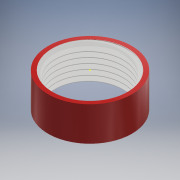
# Autodesk Inventor part: Rosca22
Saved by Autodesk Inventor 2018 (Build 220112000, 112)
## iProperties
Created: 2020-01-17
Part Number: Rosca22
Material: Generic
Document SubType Name: Modeling
Designer: Ivan
Density: 1 g/cm^3
Appearance: Default
Author: Ivan
Autodesk Inventor part; units mm, degrees
ref_plane "YZ Plane" through (0, 0, 0) normal (1, 0, 0) x (0, 1, 0)
ref_plane "XZ Plane" through (0, 0, 0) normal (0, 1, 0) x (-1, 0, 0)
ref_plane "XY Plane" through (0, 0, 0) normal (0, 0, 1) x (1, 0, 0)
sketch "Sketch1" plane through (0, 0, 0) normal (0, 0, 1) x (1, 0, 0)
  circle A0 centre (0, 0) radius 12.25
  dimension "d0" = 24.5
  constraints: 1 centre point, 1 coincident
  measures "d0" diameter of A0
extrude "Extrusion1" add sketch "Sketch1" along normal blind 10
sketch "Sketch2" plane through (0, 0, 10) normal (0, 0, 1) x (1, 0, 0)
  point P0 (0, 0)
sketch "Sketch3" plane through (0, 0, 10) normal (0, 0, 1) x (1, 0, 0)
  circle A0 centre (0, 0) radius 11
  dimension "d3" = 22
  constraints: 1 centre point, 1 coincident
  measures "d3" diameter of A0
extrude "Extrusion2" cut sketch "Sketch3" against normal through all
thread "Thread1" size "M24x1.5" class "6H" standard "ANSI Metric M Profile" full length
ref_plane "Work Plane1" through (0, 0, 10) normal (0, 0, 1) x (1, 0, 0)
ref_plane "Work Plane2" through (0, 0, 9) normal (0, 0, 1) x (1, 0, 0)
sketch "Sketch6" plane through (0, 0, 10) normal (0, 0, 1) x (1, 0, 0)
  circle A0 centre (0, 0) radius 11
  dimension "d28" = 22
  constraints: 1 centre point, 1 coincident
  measures "d28" diameter of A0
ref_plane "Work Plane3" through (0, 0, 9.5) normal (0, 0, 1) x (1, 0, 0)
thread "Thread2" size "M22x1.5" class "6H" standard "ANSI Metric M Profile" full length
sketch "Sketch12" plane through (0, 0, 0) normal (1, 0, 0) x (0, 1, 0)
  line L0 (11, 0) -> (11, 10)
  line L1 (11, 10) -> (9.8878, 10)
  line L2 (9.8878, 10) -> (9.8878, 0)
  line L3 (9.8878, 0) -> (11, 0)
  line L4 (0, -3.9629) -> (0, 12.3271) projected
  constraints: 8 end point
revolve "Revolution2" add sketch "Sketch12" angle 360 about axis through (0, 0, 0) along (0, 0, 1) separate body
sketch "Sketch11" plane through (0, 11, 0) normal (-1, 0, 0) x (0, 0, 1)
  line L0 (-0.8751, -0.076) -> (-0.7501, -0.076) construction
  line L1 (0.1249, -1.0365) -> (-0.0001, -1.2766) construction
  line L2 (-1.5001, -1.2766) -> (-1.6251, -1.0365) construction
  line L3 (-0.6251, -0.076) -> (-0.7501, 0.1641) construction
  line L4 (-0.7501, 0.1641) -> (-0.8751, -0.076) construction
  line L5 (-1.5001, -1.2766) -> (-1.3751, -1.0365) construction
  line L6 (-0.6251, -0.076) -> (-0.1251, -1.0365)
  line L7 (-1.6251, -1.0365) -> (-1.3751, -1.0365) construction
  arc A0 (-1.6251, -1.0365) -> (-1.5001, -1.1124) centre (-1.5001, -0.9714) ccw construction
  line L8 (0.1249, -1.0365) -> (-0.1251, -1.0365) construction
  line L9 (-1.5001, -1.2766) -> (-1.5001, -1.0365) construction
  line L10 (-0.0001, -1.2766) -> (-0.0001, -1.0365) construction
  line L11 (-0.7501, 0.1641) -> (-0.7501, -0.0002) construction
  line L12 (-1.5001, -1.1124) -> (-0.0001, -1.1124)
  arc A1 (-1.5001, -1.1124) -> (-1.3751, -1.0365) centre (-1.5001, -0.9714) ccw
  line L13 (-0.1251, -1.0365) -> (-0.0001, -1.2766) construction
  line L14 (-1.3751, -1.0365) -> (-0.8751, -0.076)
  line L15 (-0.0001, -0.0002) -> (-0.0001, 0.0177)
  line L16 (-0.0001, 0.0177) -> (-0.0001, -0.0002)
  line L17 (-0.0001, -0.0002) -> (0.0334, -0.0002)
  arc A2 (-0.1251, -1.0365) -> (-0.0001, -1.1124) centre (-0.0001, -0.9714) ccw
  arc A3 (-0.0001, -1.1124) -> (0.1249, -1.0365) centre (-0.0001, -0.9714) ccw construction
  arc A4 (-0.7501, -0.0002) -> (-0.8751, -0.076) centre (-0.7501, -0.1411) ccw
  arc A5 (-0.6251, -0.076) -> (-0.7501, -0.0002) centre (-0.7501, -0.1411) ccw
  line L18 (-0.7501, -0.0002) -> (-0.7501, -0.076) construction
  line L19 (-0.7501, -0.076) -> (-0.6251, -0.076) construction
  dimension "d39" = 55
  dimension "d40" = 0.2401
  dimension "d41" = 0.2401
  dimension "Sketch11_ThreadOffset" = 0
  dimension "Sketch11_MajorRadius" = 1.1122
  dimension "d44" = 1.5
  dimension "Sketch11_MinorRadius" = 0
  constraints: 40 end point, 12 point on circle, 10 parallel, 8 tangent, 6 centre point, 6 collinear, 2 midpoint, 2 point on line, 1 horizontal, 1 perpendicular, 3 other
  measures "d39" angle of L6 L14
  measures "d40" distance of L3.end L0.end
  measures "d41" distance of L1.end L10.end
  measures "Sketch11_ThreadOffset" distance between parallel lines of L15 L10
  measures "Sketch11_MajorRadius" distance from line of L12 L15.start
  measures "d44" distance from line of L1.end L9
  measures "Sketch11_MinorRadius" distance edge to line of A5 L17
coil "Coil2" sketch "Sketch11" operation cut axis through (0, 0, 0) along (0, 0, 1) pitch 1.5015 turns 8.658009 hand right bodies 2
sketch "Sketch14" plane through (0, 0, 9.5) normal (0, 0, 1) x (1, 0, 0)
  circle A0 centre (0, 0) radius 10.5
  dimension "d57" = 21
  constraints: 1 centre point, 1 coincident
  measures "d57" diameter of A0
sketch "Sketch15" plane through (0, 0, 9) normal (0, 0, 1) x (1, 0, 0)
  circle A0 centre (0, 0) radius 10
  dimension "d58" = 20
  constraints: 1 centre point, 1 coincident
  measures "d58" diameter of A0
loft "Loft2" cut profiles "Sketch6", "Sketch14", "Sketch15" bodies 1 2
equation "\"d39\" = d46"
equation "\"d40\" = 0.160083 * Sketch11_Pitch"
equation "\"d41\" = 0.160083 * Sketch11_Pitch"
equation "\"d44\" = Sketch11_Pitch"
equation "\"d15\" = 55deg"
equation "\"Sketch4_Pitch\" = 1.5"
equation "\"d46\" = 55deg"
equation "\"Sketch11_Pitch\" = 1.5"
body "Solid1"
body "Solid3"
